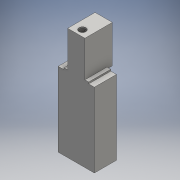
# Autodesk Inventor part: gora
Saved by Autodesk Inventor 2016 SP1 (Build 200210100, 210)
## iProperties
Created: 2019-02-21
Part Number: gora
Material: Ogólny
Document SubType Name: Modeling
Designer: Maciek
Density: 1 g/cm^3
Appearance: Domyślna
Author: Maciek
Autodesk Inventor part; units mm, degrees
ref_plane "YZ Plane" through (0, 0, 0) normal (1, 0, 0) x (0, 1, 0)
ref_plane "XZ Plane" through (0, 0, 0) normal (0, 1, 0) x (-1, 0, 0)
ref_plane "XY Plane" through (0, 0, 0) normal (0, 0, 1) x (1, 0, 0)
sketch "Szkic1" plane through (0, 0, 0) normal (0, 1, 0) x (-1, 0, 0)
  line L0 (0, 0) -> (30.6, 0)
  line L1 (30.6, 0) -> (30.6, 65.6)
  line L2 (30.6, 65.6) -> (0, 65.6)
  line L3 (0, 65.6) -> (0, 0)
  dimension "d0" = 30.6
  dimension "d1" = 65.6
  constraints: 8 end point, 2 parallel, 1 horizontal, 1 perpendicular
  measures "d0" distance of L2.end L1.end
  measures "d1" distance of L1.end L0.end
extrude "Wyciągnięcie proste1" add sketch "Szkic1" along normal blind 1.5
sketch "Szkic2" plane through (0, 1.5, 0) normal (0, 1, 0) x (1, 0, 0)
  line L0 (-30.6, 0) -> (-30.6, -65.6) construction
  line L1 (-30.6, -65.6) -> (-30.6, -62.1) construction
  line L2 (-30.6, -62.1) -> (-27.1, -62.1) construction
  line L3 (0, 0) -> (-30.6, 0) construction
  line L4 (0, 0) -> (-3.5, 0) construction
  line L5 (-3.5, 0) -> (-3.5, -3.5) construction
  line L6 (-30.6, -65.6) -> (0, -65.6) construction
  line L7 (0, -65.6) -> (-3.5, -65.6) construction
  line L8 (-3.5, -65.6) -> (-3.5, -62.1) construction
  line L9 (-3.5, -62.1) -> (0, -62.1) construction
  line L10 (0, -62.1) -> (0, -65.6) construction
  line L11 (-30.6, 0) -> (-27.1, 0) construction
  line L12 (-27.1, 0) -> (-27.1, -3.5) construction
  line L13 (-27.1, -3.5) -> (-30.6, -3.5) construction
  line L14 (-30.6, -3.5) -> (-30.6, 0) construction
  circle A0 centre (-27.1, -62.1) radius 3.4
  circle A1 centre (-3.5, -62.1) radius 3.4
  circle A2 centre (-3.5, -3.5) radius 3.4
  circle A3 centre (-27.1, -3.5) radius 3.4
  dimension "d4" = 3.5
  dimension "d5" = 3.5
  dimension "d6" = 3.5
  dimension "d7" = 3.5
  dimension "d8" = 3.5
  dimension "d9" = 3.5
  dimension "d10" = 3.5
  dimension "d11" = 3.5
  dimension "d12" = 6.8
  dimension "d13" = 6.8
  dimension "d14" = 6.8
  dimension "d15" = 6.8
  constraints: 24 end point, 4 centre point, 4 coincident, 4 parallel, 4 perpendicular, 2 horizontal, 2 point on line
  measures "d4" distance of L0.end L1.end
  measures "d5" distance of L1.end L2.end
  measures "d6" distance of L3.start L4.end
  measures "d7" distance of L4.end L5.end
  measures "d8" distance of L8.end L9.end
  measures "d9" distance of L7.end L8.end
  measures "d10" distance of L12.end L13.end
  measures "d11" distance of L11.end L12.end
  measures "d12" diameter of A0
  measures "d13" diameter of A1
  measures "d14" diameter of A2
  measures "d15" diameter of A3
extrude "Wyciągnięcie proste2" add sketch "Szkic2" along normal blind 1.5
sketch "Szkic3" plane through (-27.1, 3, 62.1) normal (0, 1, 0) x (1, 0, 0)
  circle A0 centre (23.6, 0) radius 3.4 projected
  circle A1 centre (23.6, 0) radius 1.25
  circle A2 centre (0, 0) radius 3.4 projected
  circle A3 centre (0, 0) radius 1.25
  circle A4 centre (0, 58.6) radius 3.4 projected
  circle A5 centre (0, 58.6) radius 1.25
  circle A6 centre (23.6, 58.6) radius 3.4 projected
  circle A7 centre (23.6, 58.6) radius 1.25
  point P0 (27.1, 62.1)
  dimension "d18" = 2.5
  dimension "d19" = 2.5
  dimension "d20" = 2.5
  dimension "d21" = 2.5
  constraints: 4 centre point, 4 coincident
  measures "d18" diameter of A1
  measures "d19" diameter of A3
  measures "d20" diameter of A5
  measures "d21" diameter of A7
extrude "Wyciągnięcie proste3" add sketch "Szkic3" along normal blind 2 contours A1 | A3 | A5 | A7
sketch "Szkic4" plane through (0, 0, 0) normal (0, -1, 0) x (1, 0, 0)
  line L0 (-30.6, 65.6) -> (0, 65.6) construction
  line L1 (-15.3, 65.6) -> (-25.3, 65.6) construction
  line L2 (-25.3, 65.6) -> (-5.3, 65.6)
  line L3 (-5.3, 65.6) -> (-5.3, 67.6)
  line L4 (-5.3, 67.6) -> (-25.3, 67.6)
  line L5 (-25.3, 67.6) -> (-25.3, 65.6)
  line L6 (-15.3, 67.6) -> (-21.8, 67.6) construction
  line L7 (-21.8, 67.6) -> (-8.8, 67.6)
  line L8 (-8.8, 67.6) -> (-8.8, 97.6)
  line L9 (-8.8, 97.6) -> (-21.8, 97.6)
  line L10 (-21.8, 97.6) -> (-21.8, 67.6)
  point P0 (0, 0)
  dimension "d24" = 10
  dimension "d25" = 20
  dimension "d26" = 2
  dimension "d27" = 6.5
  dimension "d28" = 13
  dimension "d29" = 30
  constraints: 20 end point, 4 parallel, 2 horizontal, 2 midpoint, 2 perpendicular, 2 point on line
  measures "d24" distance of L1.start L1.end
  measures "d25" distance of L4.end L3.end
  measures "d26" distance of L3.end L2.end
  measures "d27" distance of L6.start L6.end
  measures "d28" distance of L9.end L8.end
  measures "d29" distance of L8.end L7.end
extrude "Wyciągnięcie proste4" add sketch "Szkic4" against normal blind 1.5
sketch "Szkic6" plane through (0, 0, 0) normal (0, -1, 0) x (1, 0, 0)
  line L0 (-21.8, 97.6) -> (-8.8, 97.6) projected
  line L1 (-8.8, 97.6) -> (-21.8, 97.6)
  line L2 (-21.8, 97.6) -> (-21.8, 101.1)
  line L3 (-21.8, 101.1) -> (-8.8, 101.1)
  line L4 (-8.8, 101.1) -> (-8.8, 97.6)
  point P0 (0, 0)
  dimension "d32" = 13
  dimension "d33" = 3.5
  constraints: 8 end point, 2 parallel, 1 horizontal, 1 perpendicular
  measures "d32" distance of L2.end L3.end
  measures "d33" distance of L1.end L2.end
extrude "Wyciągnięcie proste5" add sketch "Szkic6" against normal blind 24
sketch "Szkic7" plane through (0, 1.5, 0) normal (0, 1, 0) x (1, 0, 0)
  line L0 (-21.8, -97.6) -> (-8.8, -97.6) construction
  line L1 (-21.8, -97.6) -> (-19.8, -97.6) construction
  line L2 (-19.8, -97.6) -> (-10.8, -97.6)
  line L3 (-10.8, -97.6) -> (-10.8, -95.6)
  line L4 (-10.8, -95.6) -> (-19.8, -95.6)
  line L5 (-19.8, -95.6) -> (-19.8, -97.6)
  line L6 (-21.8, -97.6) -> (-21.3, -97.6) construction
  line L7 (-21.3, -97.6) -> (-9.3, -97.6)
  line L8 (-9.3, -97.6) -> (-9.3, -94.1)
  line L9 (-9.3, -94.1) -> (-21.3, -94.1)
  line L10 (-21.3, -94.1) -> (-21.3, -97.6)
  point P0 (0, 0)
  dimension "d36" = 2
  dimension "d37" = 9
  dimension "d38" = 2
  dimension "d39" = 0.5
  dimension "d40" = 12
  dimension "d41" = 3.5
  constraints: 20 end point, 4 parallel, 2 horizontal, 2 perpendicular, 2 point on line
  measures "d36" distance of L0.start L1.end
  measures "d37" distance of L4.end L3.end
  measures "d38" distance of L3.end L2.end
  measures "d39" distance of L0.start L6.end
  measures "d40" distance of L9.end L8.end
  measures "d41" distance of L8.end L7.end
extrude "Wyciągnięcie proste6" add sketch "Szkic7" along normal blind 11 contours L7 L10 L9 L8 L3 L4 L5
sketch "Szkic8" plane through (-8.8, 24, 97.6) normal (0, 0, -1) x (-1, 0, 0)
  line L0 (11, -11.5) -> (2, -11.5) construction
  line L1 (6.5, -11.5) -> (6.5, -10.5) construction
  line L2 (6.5, -10.5) -> (6.5, -7.25) construction
  circle A0 centre (6.5, -7.25) radius 3.25
  line L3 (11, -22.5) -> (2, -22.5) construction
  line L4 (6.5, -22.5) -> (6.5, -18.25) construction
  circle A1 centre (6.5, -18.25) radius 3.25
  line L5 (9.75, -7.25) -> (9.75, -18.25)
  line L6 (3.25, -7.25) -> (3.25, -18.25)
  point P0 (-8.8, -24)
  dimension "d44" = 1
  dimension "d45" = 3.25
  dimension "d46" = 6.5
  dimension "d47" = 4.25
  dimension "d48" = 6.5
  constraints: 10 end point, 4 point on circle, 4 tangent, 3 vertical, 2 centre point, 2 coincident, 2 midpoint
  measures "d44" distance of L1.start L1.end
  measures "d45" distance of L1.end L2.end
  measures "d46" diameter of A0
  measures "d47" distance of L4.start L4.end
  measures "d48" diameter of A1
extrude "Wyciągnięcie proste7" cut sketch "Szkic8" against normal blind 11
sketch "Szkic9" plane through (0, 0, 0) normal (0, -1, 0) x (1, 0, 0)
  line L0 (-21.8, 101.1) -> (-8.8, 101.1)
  line L1 (-8.8, 101.1) -> (-8.8, 102.6)
  line L2 (-8.8, 102.6) -> (-21.8, 102.6)
  line L3 (-21.8, 102.6) -> (-21.8, 101.1)
  point P0 (0, 0)
  dimension "d51" = 13
  dimension "d52" = 1.5
  constraints: 8 end point, 2 parallel, 1 horizontal, 1 perpendicular
  measures "d51" distance of L2.end L1.end
  measures "d52" distance of L1.end L0.end
extrude "Wyciągnięcie proste8" add sketch "Szkic9" against normal blind 24
sketch "Szkic10" plane through (-21.8, 0, 102.6) normal (0, 0, 1) x (1, 0, 0)
  line L0 (13, 0) -> (0, 0) construction
  line L1 (6.5, 0) -> (6.5, 5.75) construction
  circle A0 centre (6.5, 5.75) radius 3.25
  point P0 (21.8, 0)
  dimension "d55" = 5.75
  dimension "d56" = 6.5
  constraints: 2 end point, 1 centre point, 1 coincident, 1 midpoint, 1 vertical
  measures "d55" distance of L1.start L1.end
  measures "d56" diameter of A0
extrude "Wyciągnięcie proste9" cut sketch "Szkic10" against normal blind 1.5
sketch "Szkic11" plane through (0, 24, 0) normal (0, 1, 0) x (1, 0, 0)
  line L0 (-8.8, -97.6) -> (-21.8, -97.6)
  line L1 (-21.8, -97.6) -> (-21.8, -101.1)
  line L2 (-21.8, -101.1) -> (-8.8, -101.1)
  line L3 (-8.8, -101.1) -> (-8.8, -97.6)
  point P0 (0, 0)
  dimension "d59" = 13
  dimension "d60" = 3.5
  constraints: 8 end point, 2 parallel, 1 horizontal, 1 perpendicular
  measures "d59" distance of L2.end L1.end
  measures "d60" distance of L1.end L0.end
extrude "Wyciągnięcie proste10" cut sketch "Szkic11" against normal blind 1.5
sketch "Szkic12" plane through (0, 0, 0) normal (0, -1, 0) x (1, 0, 0)
  line L0 (-30.6, 0) -> (-30.6, 65.6) projected
  line L1 (-30.6, 65.6) -> (-32.1, 65.6)
  line L2 (-32.1, 65.6) -> (-32.1, 0)
  line L3 (-32.1, 0) -> (-30.6, 0)
  line L4 (-30.6, 0) -> (-30.6, 65.6)
  point P0 (0, 0)
  dimension "d82" = 32.1
  dimension "d63" = 1.5
  dimension "d64" = 65.6
  constraints: 8 end point, 2 parallel, 1 horizontal, 1 perpendicular
  measures "d63" distance of L3.end L2.end
  measures "d64" distance of L2.end L1.end
extrude "Wyciągnięcie proste11" add sketch "Szkic12" against normal blind 19
sketch "Szkic13" plane through (-32.1, 0, 0) normal (-1, 0, 0) x (0, 0, 1)
  line L0 (65.6, 0) -> (65.6, 1.5) construction
  line L1 (65.6, 0) -> (65.6, 3) construction
  line L2 (65.6, 1.5) -> (65.6, 19) construction
  line L3 (65.6, 3) -> (0, 3) construction
  line L4 (0, 3) -> (54.3, 3) construction
  line L5 (0, 3) -> (41.7, 3) construction
  line L6 (0, 3) -> (12.7, 3) construction
  line L7 (54.3, 3) -> (58.8, 3) construction
  line L8 (41.7, 3) -> (46.2, 3) construction
  line L9 (46.2, 3) -> (37.2, 3)
  line L10 (37.2, 3) -> (37.2, 8)
  line L11 (37.2, 8) -> (46.2, 8)
  line L12 (46.2, 8) -> (46.2, 3)
  line L13 (58.8, 3) -> (49.8, 3)
  line L14 (49.8, 3) -> (49.8, 8)
  line L15 (49.8, 8) -> (58.8, 8)
  line L16 (58.8, 8) -> (58.8, 3)
  line L17 (12.7, 3) -> (18.7, 3) construction
  line L18 (18.7, 3) -> (6.7, 3)
  line L19 (6.7, 3) -> (6.7, 9)
  line L20 (6.7, 9) -> (18.7, 9)
  line L21 (18.7, 9) -> (18.7, 3)
  point P0 (0, 0)
  dimension "d67" = 3
  dimension "d68" = 54.3
  dimension "d69" = 41.7
  dimension "d70" = 12.7
  dimension "d71" = 4.5
  dimension "d72" = 4.5
  dimension "d73" = 9
  dimension "d74" = 5
  dimension "d75" = 9
  dimension "d76" = 5
  dimension "d77" = 6
  dimension "d78" = 12
  dimension "d79" = 6
  constraints: 40 end point, 7 point on line, 6 parallel, 4 horizontal, 3 perpendicular
  measures "d67" distance of L0.start L1.end
  measures "d68" distance of L3.end L4.end
  measures "d69" distance of L3.end L5.end
  measures "d70" distance of L3.end L6.end
  measures "d71" distance of L4.end L7.end
  measures "d72" distance of L5.end L8.end
  measures "d73" distance of L10.end L11.end
  measures "d74" distance of L9.end L10.end
  measures "d75" distance of L14.end L15.end
  measures "d76" distance of L13.end L14.end
  measures "d77" distance of L6.end L17.end
  measures "d78" distance of L19.end L20.end
  measures "d79" distance of L18.end L19.end
extrude "Wyciągnięcie proste12" cut sketch "Szkic13" against normal blind 1.5
sketch "Szkic14" plane through (0, 0, 0) normal (0, -1, 0) x (1, 0, 0)
  line L0 (-32.1, 65.6) -> (-32.1, 0) projected
  line L1 (-32.1, 0) -> (0, 0)
  line L2 (0, 0) -> (0, -1.5)
  line L3 (0, -1.5) -> (-32.1, -1.5)
  line L4 (-32.1, -1.5) -> (-32.1, 0)
  dimension "d82" = 32.1
  dimension "d83" = 1.5
  constraints: 8 end point, 2 parallel, 1 horizontal, 1 perpendicular
  measures "d82" distance of L2.end L3.end
  measures "d83" distance of L1.end L2.end
extrude "Wyciągnięcie proste13" add sketch "Szkic14" against normal blind 19
sketch "Szkic15" plane through (0, 0, -1.5) normal (0, 0, -1) x (-1, 0, 0)
  line L0 (32.1, 0) -> (32.1, 19) construction
  line L1 (32.1, 0) -> (32.1, 3) construction
  line L2 (6.9, 3) -> (0.1, 3) construction
  line L3 (32.1, 3) -> (0.1, 3) construction
  line L4 (0.1, 3) -> (6.7, 3) construction
  line L5 (6.7, 3) -> (20.7, 3)
  line L6 (20.7, 3) -> (20.7, 7)
  line L7 (20.7, 7) -> (6.7, 7)
  line L8 (6.7, 7) -> (6.7, 3)
  point P0 (0, 0)
  dimension "d86" = 3
  dimension "d87" = 6.6
  dimension "d88" = 14
  dimension "d89" = 4
  constraints: 14 end point, 2 parallel, 2 point on line, 1 horizontal, 1 perpendicular
  measures "d86" distance of L0.start L1.end
  measures "d87" distance of L2.end L4.end
  measures "d88" distance of L7.end L6.end
  measures "d89" distance of L6.end L5.end
extrude "Wyciągnięcie proste14" cut sketch "Szkic15" against normal blind 1.5
sketch "Szkic16" plane through (0, 0, 0) normal (0, -1, 0) x (1, 0, 0)
  line L0 (0, 65.6) -> (0, 0) projected
  line L1 (0, 65.6) -> (1.5, 65.6)
  line L2 (1.5, 65.6) -> (1.5, -1.5)
  line L3 (1.5, -1.5) -> (0, -1.5)
  line L4 (0, -1.5) -> (0, 65.6)
  dimension "d92" = 1.5
  constraints: 8 end point, 2 parallel, 1 horizontal, 1 perpendicular
  measures "d92" distance of L2.end L3.end
extrude "Wyciągnięcie proste15" add sketch "Szkic16" against normal blind 19
sketch "Szkic18" plane through (0, 0, 0) normal (0, -1, 0) x (1, 0, 0)
  line L0 (1.5, 65.6) -> (1.5, -1.5) projected
  line L1 (-5.3, 65.6) -> (-5.3, 67.6) projected
  line L2 (1.5, 65.6) -> (-5.3, 65.6)
  line L3 (-5.3, 65.6) -> (-5.3, 67.6)
  line L4 (-5.3, 67.6) -> (1.5, 67.6)
  line L5 (1.5, 67.6) -> (1.5, 65.6)
  line L6 (-25.3, 65.6) -> (-32.1, 65.6) projected
  line L7 (-21.8, 67.6) -> (-25.3, 67.6) projected
  line L8 (-32.1, 65.6) -> (-25.3, 65.6)
  line L9 (-25.3, 65.6) -> (-25.3, 67.6)
  line L10 (-25.3, 67.6) -> (-32.1, 67.6)
  line L11 (-32.1, 67.6) -> (-32.1, 65.6)
  point P0 (0, 0)
  constraints: 16 end point, 4 parallel, 2 horizontal, 2 perpendicular
extrude "Wyciągnięcie proste16" add sketch "Szkic18" against normal blind 19
sketch "Szkic19" plane through (0, 0, 0) normal (0, -1, 0) x (1, 0, 0)
  line L0 (-8.8, 97.6) -> (-8.8, 67.6) construction
  line L1 (-8.8, 67.6) -> (-7.3, 67.6) construction
  line L2 (-7.3, 67.6) -> (-7.3, 69.1) construction
  line L3 (-7.3, 69.1) -> (-8.8, 69.1) construction
  line L4 (-8.8, 69.1) -> (-8.8, 67.6) construction
  line L5 (-21.8, 67.6) -> (-21.8, 97.6) construction
  line L6 (-21.8, 67.6) -> (-23.3, 67.6) construction
  line L7 (-23.3, 67.6) -> (-23.3, 69.1) construction
  line L8 (-23.3, 69.1) -> (-21.8, 69.1) construction
  line L9 (-21.8, 69.1) -> (-21.8, 67.6) construction
  line L10 (-5.3, 67.6) -> (1.5, 67.6) construction
  line L11 (-5.3, 67.6) -> (-5.3, 69.1) construction
  line L12 (-25.3, 67.6) -> (-21.8, 67.6) construction
  line L13 (-25.3, 67.6) -> (-25.3, 69.1) construction
  line L14 (-5.3, 69.1) -> (-3.8, 69.1) construction
  line L15 (-3.8, 69.1) -> (-3.8, 67.6) construction
  line L16 (-3.8, 67.6) -> (-5.3, 67.6) construction
  line L17 (-5.3, 67.6) -> (-5.3, 69.1) construction
  line L18 (-25.3, 69.1) -> (-26.8, 69.1) construction
  line L19 (-26.8, 69.1) -> (-26.8, 67.6) construction
  line L20 (-26.8, 67.6) -> (-25.3, 67.6) construction
  line L21 (-25.3, 67.6) -> (-25.3, 69.1) construction
  line L22 (-8.8, 67.6) -> (-8.8, 102.6) construction
  line L23 (-8.8, 102.6) -> (-7.3, 102.6) construction
  line L24 (-21.8, 102.6) -> (-21.8, 67.6) construction
  line L25 (-21.8, 102.6) -> (-23.3, 102.6) construction
  line L26 (-7.3, 102.6) -> (-8.8, 102.6)
  line L27 (-8.8, 102.6) -> (-8.8, 69.1)
  line L28 (-8.8, 69.1) -> (-7.3, 69.1)
  line L29 (-7.3, 69.1) -> (-7.3, 102.6)
  line L30 (-23.3, 102.6) -> (-21.8, 102.6)
  line L31 (-21.8, 102.6) -> (-21.8, 69.1)
  line L32 (-21.8, 69.1) -> (-23.3, 69.1)
  line L33 (-23.3, 69.1) -> (-23.3, 102.6)
  line L34 (-8.8, 67.6) -> (-5.3, 67.6) projected
  line L35 (-3.8, 69.1) -> (-8.8, 69.1)
  line L36 (-8.8, 69.1) -> (-8.8, 67.6)
  line L37 (-8.8, 67.6) -> (-3.8, 67.6)
  line L38 (-3.8, 67.6) -> (-3.8, 69.1)
  line L39 (-26.8, 67.6) -> (-21.8, 67.6)
  line L40 (-21.8, 67.6) -> (-21.8, 69.1)
  line L41 (-21.8, 69.1) -> (-26.8, 69.1)
  line L42 (-26.8, 69.1) -> (-26.8, 67.6)
  point P0 (0, 0)
  dimension "d97" = 1.5
  dimension "d98" = 1.5
  dimension "d99" = 1.5
  dimension "d100" = 1.5
  dimension "d101" = 1.5
  dimension "d102" = 1.5
  dimension "d103" = 1.5
  dimension "d104" = 1.5
  dimension "d105" = 1.5
  dimension "d106" = 1.5
  constraints: 72 end point, 16 parallel, 10 horizontal, 8 perpendicular, 2 vertical
  measures "d97" distance of L3.end L2.end
  measures "d98" distance of L2.end L1.end
  measures "d99" distance of L7.end L8.end
  measures "d100" distance of L6.end L7.end
  measures "d101" distance of L15.end L16.end
  measures "d102" distance of L14.end L15.end
  measures "d103" distance of L20.end L19.end
  measures "d104" distance of L19.end L18.end
  measures "d105" distance of L22.end L23.end
  measures "d106" distance of L24.start L25.end
extrude "Wyciągnięcie proste17" add sketch "Szkic19" against normal blind 24 contours L29 L28 L27 L26 | L30 L31 L32 L33
sketch "Szkic20" plane through (0, 0, 0) normal (0, -1, 0) x (1, 0, 0)
  line L0 (-25.3, 67.6) -> (-21.8, 67.6) construction
  line L1 (-25.3, 67.6) -> (-26.8, 67.6) construction
  line L2 (-26.8, 67.6) -> (-26.8, 69.1) construction
  line L3 (-26.8, 69.1) -> (-25.3, 69.1) construction
  line L4 (-25.3, 69.1) -> (-25.3, 67.6) construction
  line L5 (-8.8, 67.6) -> (-5.3, 67.6) construction
  line L6 (-5.3, 67.6) -> (-3.8, 67.6) construction
  line L7 (-3.8, 67.6) -> (-3.8, 69.1) construction
  line L8 (-3.8, 69.1) -> (-5.3, 69.1) construction
  line L9 (-5.3, 69.1) -> (-5.3, 67.6) construction
  line L10 (-26.8, 69.1) -> (-21.8, 69.1)
  line L11 (-21.8, 69.1) -> (-21.8, 67.6)
  line L12 (-21.8, 67.6) -> (-26.8, 67.6)
  line L13 (-26.8, 67.6) -> (-26.8, 69.1)
  line L14 (-8.8, 67.6) -> (-3.8, 67.6)
  line L15 (-3.8, 67.6) -> (-3.8, 69.1)
  line L16 (-3.8, 69.1) -> (-8.8, 69.1)
  line L17 (-8.8, 69.1) -> (-8.8, 67.6)
  point P0 (0, 0)
  dimension "d109" = 1.5
  dimension "d110" = 1.5
  dimension "d111" = 1.5
  dimension "d112" = 1.5
  constraints: 32 end point, 8 parallel, 4 horizontal, 4 perpendicular
  measures "d109" distance of L2.end L3.end
  measures "d110" distance of L1.end L2.end
  measures "d111" distance of L8.end L7.end
  measures "d112" distance of L7.end L6.end
extrude "Wyciągnięcie proste18" add sketch "Szkic20" against normal blind 19
sketch "Szkic21" plane through (0, 19, 0) normal (0, 1, 0) x (1, 0, 0)
  line L0 (-5.3, -65.6) -> (-5.3, -67.6) projected
  line L1 (-25.3, -67.6) -> (-5.3, -67.6)
  line L2 (0, -65.6) -> (-5.3, -65.6) projected
  line L3 (-5.3, -67.6) -> (-5.3, -65.6)
  line L4 (-5.3, -65.6) -> (0, -65.6)
  line L5 (0, 0) -> (0, -65.6) projected
  line L6 (0, -65.6) -> (0, 0)
  line L7 (-30.6, -65.6) -> (-30.6, 0) projected
  line L8 (0, 0) -> (-30.6, 0)
  line L9 (-30.6, 0) -> (-30.6, -65.6)
  line L10 (-25.3, -67.6) -> (-25.3, -65.6) projected
  line L11 (-30.6, -65.6) -> (-25.3, -65.6)
  line L12 (-25.3, -65.6) -> (-25.3, -67.6)
  line L13 (-30.6, -65.6) -> (-29.1, -65.6) construction
  line L14 (-29.1, -65.6) -> (-29.1, -64.1) construction
  line L15 (-29.1, -64.1) -> (-30.6, -64.1) construction
  line L16 (-30.6, -64.1) -> (-30.6, -65.6) construction
  line L17 (-30.6, 0) -> (-29.1, 0) construction
  line L18 (-29.1, 0) -> (-29.1, -1.5) construction
  line L19 (-29.1, -1.5) -> (-30.6, -1.5) construction
  line L20 (-30.6, -1.5) -> (-30.6, 0) construction
  line L21 (0, 0) -> (-1.5, 0) construction
  line L22 (-1.5, 0) -> (-1.5, -1.5) construction
  line L23 (-1.5, -1.5) -> (0, -1.5) construction
  line L24 (0, -1.5) -> (0, 0) construction
  line L25 (0, -65.6) -> (-1.5, -65.6) construction
  line L26 (-1.5, -65.6) -> (-1.5, -64.1) construction
  line L27 (-1.5, -64.1) -> (0, -64.1) construction
  line L28 (0, -64.1) -> (0, -65.6) construction
  line L29 (-5.3, -65.6) -> (-6.8, -65.6) construction
  line L30 (-6.8, -65.6) -> (-6.8, -64.1) construction
  line L31 (-6.8, -64.1) -> (-5.3, -64.1) construction
  line L32 (-5.3, -64.1) -> (-5.3, -65.6) construction
  line L33 (-5.3, -67.6) -> (-6.8, -67.6) construction
  line L34 (-6.8, -67.6) -> (-6.8, -66.1) construction
  line L35 (-6.8, -66.1) -> (-5.3, -66.1) construction
  line L36 (-5.3, -66.1) -> (-5.3, -67.6) construction
  line L37 (-21.8, -67.6) -> (-25.3, -67.6) construction
  line L38 (-25.3, -67.6) -> (-23.8, -67.6) construction
  line L39 (-23.8, -67.6) -> (-23.8, -66.1) construction
  line L40 (-23.8, -66.1) -> (-25.3, -66.1) construction
  line L41 (-25.3, -66.1) -> (-25.3, -67.6) construction
  line L42 (-25.3, -65.6) -> (-23.8, -65.6) construction
  line L43 (-23.8, -65.6) -> (-23.8, -64.1) construction
  line L44 (-23.8, -64.1) -> (-25.3, -64.1) construction
  line L45 (-25.3, -64.1) -> (-25.3, -65.6) construction
  line L46 (-29.1, -64.1) -> (-29.1, -1.5)
  line L47 (-29.1, -1.5) -> (-1.5, -1.5)
  line L48 (-1.5, -1.5) -> (-1.5, -64.1)
  line L49 (-1.5, -64.1) -> (-6.8, -64.1)
  line L50 (-6.8, -64.1) -> (-6.8, -66.1)
  line L51 (-6.8, -66.1) -> (-23.8, -66.1)
  line L52 (-23.8, -66.1) -> (-23.8, -64.1)
  line L53 (-23.8, -64.1) -> (-29.1, -64.1)
  dimension "d115" = 1.5
  dimension "d116" = 1.5
  dimension "d117" = 1.5
  dimension "d118" = 1.5
  dimension "d119" = 1.5
  dimension "d120" = 1.5
  dimension "d121" = 1.5
  dimension "d122" = 1.5
  dimension "d123" = 1.5
  dimension "d124" = 1.5
  dimension "d125" = 1.5
  dimension "d126" = 1.5
  dimension "d127" = 1.5
  dimension "d128" = 1.5
  dimension "d129" = 1.5
  dimension "d130" = 1.5
  constraints: 96 end point, 18 equal length, 13 perpendicular, 9 horizontal
  measures "d115" distance of L15.end L14.end
  measures "d116" distance of L14.end L13.end
  measures "d117" distance of L18.end L19.end
  measures "d118" distance of L17.end L18.end
  measures "d119" distance of L23.end L22.end
  measures "d120" distance of L22.end L21.end
  measures "d121" distance of L26.end L27.end
  measures "d122" distance of L25.end L26.end
  measures "d123" distance of L30.end L31.end
  measures "d124" distance of L29.end L30.end
  measures "d125" distance of L34.end L35.end
  measures "d126" distance of L33.end L34.end
  measures "d127" distance of L40.end L39.end
  measures "d128" distance of L39.end L38.end
  measures "d129" distance of L44.end L43.end
  measures "d130" distance of L43.end L42.end
extrude "Wyciągnięcie proste19" add sketch "Szkic21" against normal blind 2
sketch "Szkic22" plane through (0, 19, 0) normal (0, 1, 0) x (1, 0, 0)
  line L0 (1.5, -67.6) -> (1.5, 1.5) projected
  line L1 (1.5, -67.6) -> (1.5, 1.5)
  line L2 (1.5, 1.5) -> (-32.1, 1.5) projected
  line L3 (1.5, 1.5) -> (-32.1, 1.5)
  line L4 (-32.1, -67.6) -> (-26.8, -67.6) projected
  line L5 (-32.1, 1.5) -> (-32.1, -67.6)
  line L6 (-32.1, -67.6) -> (-26.8, -67.6)
  line L7 (-26.8, -69.1) -> (-23.3, -69.1) projected
  line L8 (-26.8, -67.6) -> (-26.8, -69.1)
  line L9 (-7.3, -69.1) -> (-3.8, -69.1) projected
  line L10 (-26.8, -69.1) -> (-3.8, -69.1)
  line L11 (-3.8, -69.1) -> (-3.8, -67.6)
  line L12 (-3.8, -67.6) -> (1.5, -67.6) projected
  line L13 (-3.8, -67.6) -> (1.5, -67.6)
  point P0 (0, 0)
  constraints: 16 end point, 6 perpendicular, 1 collinear, 1 point on line, 1 vertical
extrude "Wyciągnięcie proste20" add sketch "Szkic22" along normal blind 1.5
sketch "Szkic23" plane through (0, 24, 0) normal (0, 1, 0) x (1, 0, 0)
  line L0 (-21.8, -101.1) -> (-21.8, -97.6) projected
  line L1 (-8.8, -67.6) -> (-8.8, -69.1) projected
  line L2 (-21.8, -101.1) -> (-8.8, -101.1)
  line L3 (-8.8, -101.1) -> (-8.8, -69.1)
  line L4 (-8.8, -69.1) -> (-21.8, -69.1)
  line L5 (-21.8, -69.1) -> (-21.8, -101.1)
  line L6 (-21.8, -101.1) -> (-20.3, -101.1) construction
  line L7 (-20.3, -101.1) -> (-20.3, -99.6) construction
  line L8 (-20.3, -99.6) -> (-21.8, -99.6) construction
  line L9 (-21.8, -99.6) -> (-21.8, -101.1) construction
  line L10 (-8.8, -69.1) -> (-10.3, -69.1) construction
  line L11 (-21.8, -69.1) -> (-8.8, -69.1) construction
  line L12 (-20.3, -99.6) -> (-10.3, -99.6)
  line L13 (-10.3, -99.6) -> (-10.3, -69.1)
  line L14 (-10.3, -69.1) -> (-20.3, -69.1)
  line L15 (-20.3, -69.1) -> (-20.3, -99.6)
  point P0 (0, 0)
  dimension "d135" = 1.5
  dimension "d136" = 1.5
  dimension "d137" = 1.5
  constraints: 26 end point, 6 parallel, 3 horizontal, 3 perpendicular, 1 point on line
  measures "d135" distance of L8.end L7.end
  measures "d136" distance of L7.end L6.end
  measures "d137" distance of L1.end L10.end
extrude "Wyciągnięcie proste21" add sketch "Szkic23" against normal blind 1.5 contours L0 L5 L4 L15 L12 L13 L3 L2
sketch "Szkic24" plane through (0, 24, 0) normal (0, 1, 0) x (1, 0, 0)
  line L0 (-23.3, -69.1) -> (-23.3, -102.6) projected
  line L1 (-23.3, -69.1) -> (-7.3, -69.1)
  line L2 (-7.3, -69.1) -> (-7.3, -67.6)
  line L3 (-7.3, -67.6) -> (-23.3, -67.6)
  line L4 (-23.3, -67.6) -> (-23.3, -69.1)
  point P0 (0, 0)
  dimension "d140" = 16
  dimension "d141" = 1.5
  constraints: 8 end point, 2 parallel, 1 horizontal, 1 perpendicular
  measures "d140" distance of L3.end L2.end
  measures "d141" distance of L2.end L1.end
extrude "Wyciągnięcie proste22" add sketch "Szkic24" against normal blind 3.5
sketch "Szkic25" plane through (0, 24, 0) normal (0, 1, 0) x (1, 0, 0)
  line L0 (-7.3, -102.6) -> (-7.3, -69.1) projected
  line L1 (-23.3, -69.1) -> (-23.3, -67.6) projected
  line L2 (-7.3, -102.6) -> (-23.3, -102.6)
  line L3 (-23.3, -102.6) -> (-23.3, -67.6)
  line L4 (-23.3, -67.6) -> (-7.3, -67.6)
  line L5 (-7.3, -67.6) -> (-7.3, -102.6)
  point P0 (0, 0)
  constraints: 8 end point, 2 parallel, 1 horizontal, 1 perpendicular
extrude "Wyciągnięcie proste23" add sketch "Szkic25" along normal blind 1.5
sketch "Szkic26" plane through (0, 20.5, 0) normal (0, 1, 0) x (1, 0, 0)
  line L0 (1.5, -67.6) -> (1.5, 1.5) construction
  line L1 (1.5, 1.5) -> (1.5, -0.3) construction
  line L2 (1.5, -0.3) -> (1.5, -25.3) construction
  line L3 (1.5, -0.3) -> (1.5, -48.3) construction
  line L4 (1.5, -48.3) -> (0, -48.3) construction
  line L5 (0, -48.3) -> (-7, -48.3)
  line L6 (-7, -48.3) -> (-7, -25.3)
  line L7 (-7, -25.3) -> (0, -25.3)
  line L8 (0, -25.3) -> (0, -48.3)
  point P0 (0, 0)
  dimension "d146" = 1.8
  dimension "d147" = 25
  dimension "d148" = 48
  dimension "d149" = 7
  constraints: 16 end point, 3 point on line, 2 horizontal, 2 parallel, 1 perpendicular
  measures "d146" distance of L0.end L1.end
  measures "d147" distance of L1.end L2.end
  measures "d148" distance of L1.end L3.end
  measures "d149" distance of L6.end L7.end
extrude "Wyciągnięcie proste24" cut sketch "Szkic26" against normal blind 5
